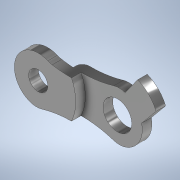
# Autodesk Inventor part: Part6
Saved by Autodesk Inventor 2021 (Build 250183000, 183)
## iProperties
Created: 2020-11-21
Part Number: Part6
Material: Nickel-Copper Alloy 400
Document SubType Name: Modeling
Designer: pedro
Density: 8.83 g/cm^3
Appearance: Cromado - Preto polido
Author: pedro
Autodesk Inventor part; units mm, degrees
ref_plane "YZ Plane" through (0, 0, 0) normal (1, 0, 0) x (0, 1, 0)
ref_plane "XZ Plane" through (0, 0, 0) normal (0, 1, 0) x (-1, 0, 0)
ref_plane "XY Plane" through (0, 0, 0) normal (0, 0, 1) x (1, 0, 0)
sketch "Sketch1" plane through (0, 0, 0) normal (0, 0, 1) x (1, 0, 0)
  arc A0 (-5.6835, 2.2943) -> (-7.6273, -2.3122) centre (-6.6766, 0) ccw
  arc A1 (-5.2258, 2.1583) -> (0.2129, 2.4842) centre (-3.2055, 13.987) ccw
  line L0 (-6.6766, 2.5) -> (-6.6766, -2.5) construction
  arc A2 (-5.6835, 2.2943) -> (-5.2258, 2.1583) centre (-4.8891, 4.1298) ccw
  arc A3 (1.5395, -2.4196) -> (1.4069, 2.4672) centre (0.5964, 0) ccw
  arc A4 (1.4069, 2.4672) -> (0.2129, 2.4842) centre (0.7827, 0.5671) ccw
  line L1 (0.5964, 2.5969) -> (0.5964, -2.5969) construction
  arc A5 (0.1965, -2.4587) -> (-6.2967, -2.3795) centre (-3.1776, -12.8694) ccw
  arc A6 (-7.6273, -2.3122) -> (-6.2967, -2.3795) centre (-6.8667, -0.4624) ccw
  arc A7 (0.1965, -2.4587) -> (1.5395, -2.4196) centre (0.8132, -0.5562) ccw
  circle A8 centre (-6.6766, 0) radius 1
  circle A9 centre (0.5964, 0) radius 1.5
  line L2 (1.4069, 2.4672) -> (2.7069, 4.2755)
  line L3 (3.1306, 0.5671) -> (4.6306, 2.3807)
  arc A10 (4.6306, 2.3807) -> (2.7069, 4.2755) centre (1.4088, 1.0336) ccw
  line L4 (-3.2055, 1.987) -> (-3.2055, -1.9256) construction
  line L5 (-3.2055, 1.987) -> (-3.2055, -1.9256) construction
  arc A11 (-3.2055, -1.9256) -> (-3.2055, 1.987) centre (-7.3367, 0.0307) ccw
  point P0 (0, 0)
  dimension "d0" = 5
  dimension "d1" = 12
  dimension "d2" = 2
  dimension "d3" = 2
  dimension "d5" = 2
  dimension "d6" = 2
  dimension "d7" = 3
  dimension "d8" = 1.5
  dimension "d9" = 1.3
  constraints: 29 point on circle, 12 centre point, 12 end point, 8 tangent, 4 vertical, 2 coincident, 1 equal radius
  measures "d0" diameter of A0
  measures "d1" radius of A1
  measures "d2" radius of A2
  measures "d3" radius of A4
  measures "d5" radius of A6
  measures "d6" diameter of A8
  measures "d7" diameter of A9
  measures "d8" horizontal distance of L3.start L3.end
  measures "d9" horizontal distance of L2.start L2.end
extrude "Extrusion1" add sketch "Sketch1" along normal blind 1 contours A2 A1 A11 A5 A6 A0
extrude "Extrusion2" add sketch "Sketch1" against normal blind 1 contours A1 A4 A3 A7 A5 A11
extrude "Extrusion3" add sketch "Sketch1" against normal blind 1 contours L2 A10 L3 A3
sketch "Esboço2" plane through (0, 0, 0) normal (0, 0, -1) x (-1, 0, 0)
  line L0 (4.0311, 2.0155) -> (4.0311, -1.9589)
  arc A0 (3.2055, 1.987) -> (3.2055, -1.9256) centre (7.3367, 0.0307) ccw projected
  arc A1 (3.2055, 1.987) -> (3.2055, -1.9256) centre (7.3367, 0.0307) ccw
  arc A2 (3.2055, 1.987) -> (5.2258, 2.1583) centre (3.2055, 13.987) ccw projected
  arc A3 (6.2967, -2.3795) -> (3.2055, -1.9256) centre (3.1776, -12.8694) ccw projected
  point P0 (0, 0)
  constraints: 2 end point, 2 point on circle, 1 centre point, 1 vertical
extrude "Extrusão4" add sketch "Esboço2" along normal blind 1
fillet "Arredondamento1" radius 0.7 1 edges at (-4.0311, 0.0283, -1)
body "Solid1"
